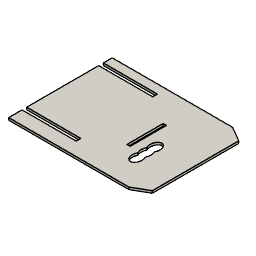
second_chassis (Autodesk Fusion 360 design; units mm, degrees)
part number: 2026-06-29-19-26-32-904
Autodesk Fusion 360 part; units mm, degrees
sketch "Sketch1" plane through (0, 0, 0) normal (0, 0, 1) x (1, 0, 0)
  line L0 (0, 0) -> (0, 230)
  line L1 (0, 230) -> (267, 230)
  line L2 (267, 230) -> (300, 210.9474)
  line L3 (300, 19.0526) -> (267, 0)
  line L4 (267, 0) -> (0, 0)
  line L5 (300, 210.9474) -> (300, 19.0526)
  dimension "d1" = 230
  dimension "d2" = 267
  dimension "d3" = 33
  dimension "d4" = 150
  dimension "d5" = 150
  constraint coincident L0.start L4.end
  constraint vertical L0
  constraint perpendicular L0 L1
  constraint perpendicular L0 L4
  constraint vertical L5
  constraint equal L1 L4
  measures "d1" distance of L0.start L0.end
  measures "d2" distance of L0.start L3.end
  measures "d3" horizontal distance of L3.start L3.end
  measures "d4" angle of L3 L4
  measures "d5" angle of L1 L2
extrude "Extrude1" add sketch "Sketch1" along normal blind 5
sketch "Sketch2" plane through (0, 0, 5) normal (0, 0, 1) x (-1, 0, 0)
  line L0 (-300, -210.9474) -> (-267, -230)
  line L1 (-267, -230) -> (0, -230)
  line L2 (0, -230) -> (0, 0)
  line L3 (0, 0) -> (-267, 0)
  line L4 (-267, 0) -> (-300, -19.0526)
  line L5 (-300, -19.0526) -> (-300, -210.9474)
  ellipse E0 centre (-219.2825, -65.8758) end of major axis (-229.95, -65.8758) minor radius 15
  line L6 (-208.6151, -65.8758) -> (-229.95, -65.8758) construction
  line L7 (-219.2825, -50.8758) -> (-219.2825, -80.8758) construction
  dimension "d8" = 30
  constraint coincident E0 L6.start
  constraint coincident E0 L6.end
  constraint coincident E0 L7.start
  constraint coincident E0 L7.end
  constraint horizontal L6
extrude "Extrude2" cut sketch "Sketch2" against normal through all contours E0
pattern_linear "R-Pattern1" count 3 spacing 20 along (0, 1, 0) of "Extrude2"
sketch "Sketch3" plane through (0, 0, 5) normal (0, 0, 1) x (-1, 0, 0)
  ellipse E0 centre (-219.2825, -85.8758) end of major axis (-219.2825, -100.8758) minor radius 10.6675 (-227.2336, -75.8758) -> (-227.2336, -95.8758) ccw
  ellipse E1 centre (-219.2825, -65.8758) end of major axis (-219.2825, -80.8758) minor radius 10.6675 (-211.3315, -75.8758) -> (-227.2336, -75.8758) ccw
  ellipse E2 centre (-219.2825, -85.8758) end of major axis (-219.2825, -100.8758) minor radius 10.6675 (-211.3315, -95.8758) -> (-211.3315, -75.8758) ccw
  ellipse E3 centre (-219.2825, -105.8758) end of major axis (-219.2825, -120.8758) minor radius 10.6675 (-227.2336, -95.8758) -> (-211.3315, -95.8758) ccw
  line L0 (-300, -210.9474) -> (-267, -230)
  line L1 (-267, -230) -> (0, -230)
  line L2 (0, -230) -> (0, 0)
  line L3 (0, 0) -> (-267, 0)
  line L4 (-267, 0) -> (-300, -19.0526)
  line L5 (-300, -19.0526) -> (-300, -210.9474)
  line L6 (0, -40) -> (-120, -40)
  line L7 (-120, -40) -> (-120, -30)
  line L8 (-120, -30) -> (0, -30)
  line L9 (0, -30) -> (0, -40)
  line L10 (0, -210) -> (-120, -210)
  line L11 (-120, -210) -> (-120, -200)
  line L12 (-120, -200) -> (0, -200)
  line L13 (0, -200) -> (0, -210)
  line L14 (-183, -210) -> (-190, -210)
  line L15 (-190, -210) -> (-190, -30)
  line L16 (-190, -30) -> (-183, -30)
  line L17 (-183, -30) -> (-183, -210)
  line L18 (-190, -160) -> (-183, -160)
  line L19 (-190, -80) -> (-183, -80)
  dimension "d15" = 30
  dimension "d16" = 10
  dimension "d18" = 120
  dimension "d19" = 20
  dimension "d21" = 10
  dimension "d22" = 180
  dimension "d26" = 30
  dimension "d30" = 180
  dimension "d31" = 7
  dimension "d33" = 70
  dimension "d34" = 30
  dimension "d35" = 110
  dimension "d36" = 80
  dimension "d37" = 20
  dimension "d38" = 50
  constraint horizontal L6
  constraint vertical L7
  constraint horizontal L8
  constraint vertical L9
  constraint horizontal L10
  constraint vertical L11
  constraint horizontal L12
  constraint vertical L13
  constraint coincident L2 L10.start
  constraint equal L6 L12
  constraint horizontal L14
  constraint vertical L15
  constraint horizontal L16
  constraint vertical L17
  constraint coincident L15 L18.start
  constraint coincident L17 L18.end
  constraint perpendicular L15 L18
  constraint coincident L15 L19.start
  constraint coincident L17 L19.end
  constraint perpendicular L15 L19
  measures "d15" distance of L3 L8
  measures "d16" distance of L6.end L7.end
  measures "d18" distance of L6.start L6.end
  measures "d19" distance of L1 L10
  measures "d21" distance of L10.end L11.end
  measures "d22" distance of L8 L10
  measures "d26" distance of L3 L8
  measures "d30" distance of L5 L7
  measures "d31" distance of L14.start L14.end
  measures "d33" distance of L7 L15
  measures "d34" distance of L3 L16
  measures "d35" distance of L5 L15
  measures "d36" distance of L18 L19
  measures "d37" distance of L1 L14
  measures "d38" distance of L14 L18
extrude "Extrude4" cut sketch "Sketch3" against normal through all contours L2 L10 L11 L12 L13 | L2 L6 L7 L8 L9
extrude "Extrude6" cut sketch "Sketch3" against normal through all contours L15 L17 L18 L19
